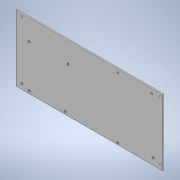
# Autodesk Inventor part: 20220620_知能ロボットコンテスト二階部分
Saved by Autodesk Inventor 2020 (Build 240168000, 168)
## iProperties
Created: 2022-06-20
Part Number: 20220620_知能ロボットコンテスト二階部分
Material: 一般
Document SubType Name: Modeling
Designer: Naggy
Density: 1 g/cm^3
Appearance: 既定
Author: Naggy
Autodesk Inventor part; units mm, degrees
ref_plane "YZ Plane" through (0, 0, 0) normal (1, 0, 0) x (0, 1, 0)
ref_plane "XZ Plane" through (0, 0, 0) normal (0, 1, 0) x (-1, 0, 0)
ref_plane "XY Plane" through (0, 0, 0) normal (0, 0, 1) x (1, 0, 0)
sketch "スケッチ1" plane through (0, 0, 0) normal (0, 0, 1) x (1, 0, 0)
  line L0 (-100, -45) -> (100, -45)
  line L1 (100, -45) -> (100, 45)
  line L2 (100, 45) -> (-100, 45)
  line L3 (-100, 45) -> (-100, -45)
  line L4 (-100, -45) -> (100, 45) construction
  line L5 (100, -45) -> (-100, 45) construction
  point P0 (0, 0)
  dimension "d0" = 90
  dimension "d1" = 200
  constraints: 12 end point, 2 midpoint, 2 parallel, 1 horizontal, 1 perpendicular
  measures "d0" distance between parallel lines of L0 L2
  measures "d1" distance between parallel lines of L3 L1
extrude "押し出し1" add sketch "スケッチ1" along normal blind 1.5
sketch "スケッチ2" plane through (0, 0, 1.5) normal (0, 0, 1) x (1, 0, 0)
  line L0 (100, -45) -> (100, 45) projected
  line L1 (-100, -45) -> (100, -45) projected
  point P0 (0, 0)
  point P1 (97, 41)
  point P2 (97, -39)
  dimension "d4" = 3
  dimension "d5" = 3
  dimension "d6" = 6
  dimension "d7" = 86
  measures "d4" distance from line of point (97, 41) L0
  measures "d5" distance from line of L0 point (97, -39)
  measures "d6" distance from line of point (97, -39) L1
  measures "d7" distance from line of point (97, 41) L1
hole "穴1" at (97, 41, 1.5) at (97, -39, 1.5) direction (0, 0, -1) diameter 2.5 depth 8.8 tip angle 118
sketch "スケッチ3" plane through (0, 0, 1.5) normal (0, 0, 1) x (1, 0, 0)
  line L0 (-100, 45) -> (-100, -45) projected
  line L1 (-100, -45) -> (100, -45) projected
  point P0 (0, 0)
  point P1 (-92, 41)
  point P2 (-92, -38)
  dimension "d15" = 8
  dimension "d16" = 8
  dimension "d17" = 7
  dimension "d18" = 86
  measures "d15" distance from line of point (-92, 41) L0
  measures "d16" distance from line of point (-92, -38) L0
  measures "d17" distance from line of point (-92, -38) L1
  measures "d18" distance from line of point (-92, 41) L1
hole "穴2" at (-92, 41, 1.5) at (-92, -38, 1.5) direction (0, 0, -1) diameter 2.5 depth 8.8 tip angle 118
sketch "スケッチ4" plane through (0, 0, 1.5) normal (0, 0, 1) x (1, 0, 0)
  circle A0 centre (97, -39) radius 1.25 projected
  line L0 (-100, -45) -> (100, -45) projected
  point P0 (0, 0)
  point P1 (85.0067, 38.82)
  point P2 (87, -36.11)
  dimension "d26" = 10
  dimension "d27" = 8.89
  dimension "d28" = 74.93
  measures "d26" horizontal distance of point (87, -36.11) A0.centre
  measures "d27" distance from line of point (87, -36.11) L0
  measures "d28" vertical distance of point (85.007, 38.82) point (87, -36.11)
hole "穴3" at (85.0067, 38.82, 1.5) at (87, -36.11, 1.5) direction (0, 0, -1) diameter 2.459 depth 8.8 tip angle 118 thread size "M3x0.5" class "6H" standard "ANSI Metric M Profile"
sketch "スケッチ5" plane through (0, 0, 1.5) normal (0, 0, 1) x (1, 0, 0)
  circle A0 centre (87, -36.11) radius 1.2295 projected
  line L0 (-100, -45) -> (100, -45) projected
  point P0 (0, 0)
  point P1 (38.74, -42.46)
  point P2 (38.74, 40.09)
  dimension "d36" = 48.26
  dimension "d37" = 2.54
  dimension "d38" = 82.55
  measures "d36" horizontal distance of point (38.74, -42.46) A0.centre
  measures "d37" distance from line of point (38.74, -42.46) L0
  measures "d38" distance of point (38.74, 40.09) point (38.74, -42.46)
hole "穴4" at (38.74, -42.46, 1.5) at (38.74, 40.09, 1.5) direction (0, 0, -1) diameter 2.459 depth 8.8 tip angle 118 thread size "M3x0.5" class "6H" standard "ANSI Metric M Profile"
sketch "スケッチ6" plane through (0, 0, 1.5) normal (0, 0, 1) x (1, 0, 0)
  line L0 (-100, -45) -> (100, -45) projected
  circle A0 centre (-92, -38) radius 1.25 projected
  point P0 (0, 0)
  point P1 (-82.2925, 16.5)
  point P2 (-29.1034, 16.5)
  point P3 (-82, -41.5)
  point P4 (-33, -41.5)
  dimension "d46" = 3.5
  dimension "d47" = 10
  dimension "d48" = 49
  dimension "d49" = 3.5
  dimension "d50" = 58
  dimension "d51" = 58
  measures "d46" distance from line of point (-82, -41.5) L0
  measures "d47" horizontal distance of point (-82, -41.5) A0.centre
  measures "d48" distance of point (-33, -41.5) point (-82, -41.5)
  measures "d49" distance from line of point (-33, -41.5) L0
  measures "d50" vertical distance of point (-82.292, 16.5) point (-82, -41.5)
  measures "d51" vertical distance of point (-29.103, 16.5) point (-33, -41.5)
hole "穴5" at (-82.2925, 16.5, 1.5) at (-29.1034, 16.5, 1.5) at (-82, -41.5, 1.5) at (-33, -41.5, 1.5) direction (0, 0, -1) diameter 2.459 depth 8.8 tip angle 118 thread size "M3x0.5" class "6H" standard "ANSI Metric M Profile"
